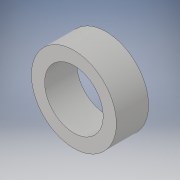
# Autodesk Inventor part: C-TFK10_c
Saved by Autodesk Inventor 2021 (Build 250183000, 183)
## iProperties
Created: 2023-03-01
Part Number: C-TFK10_c
Material: Generic
Catalog Web Link: www.cadenas.de
Description: C-TFK_c-Economy Support Units Fixed Side Round
Vendor: MISUMI
Document SubType Name: Modeling
Designer: psAdmin
Manufacturer: MISUMI
Mass: 0.476246 g
Surface Area: 5.9651 cm^2
Volume: 0.476246 cm^3
Density: 1 g/cm^3
Appearance: PSOLRGB-175-175-175
Category: PARTsolutions
Company: MISUMI
PSOL_IDENT_0: {$CADENAS_DATA/23d-libs/misumi/metric/09_ball_screws/c_tfk/c_tfk_collar.prj},161 {VTYP=3D},{NB=C-TFK
PSOL_IDENT_1: 10_c},{LINA=C-TFK10},{NN=C-TFK_c},{DATE=14.09.2022 01:48:01},{GEOMDATE=16.11.2021 00:24:26},{VERSION=
PSOL_IDENT_2: },{LINEID=100},{WBVAR=SET},{WBNUMERIC=}  {NB=C-TFK10_c},{LINA=C-TFK10},{KT=DUMMY},{PN=C-TFK10},{TYPE=
PSOL_IDENT_3: C-TFK},{NO=10},{SET=},{DD=10},{L=27},{H=10},{F=17},{E=29.5},{D=34},{A=52},{PCD=42},{B=42},{L1=7.5},{
PSOL_IDENT_4: T1=5.0},{DD1=4.5},{DD2=8.0},{LL=4.0},{M=M10x1.0},{T=16},{SID=14.0},{ACD=14.5},{ACV=10},{ACL=5.5}
NB: C-TFK10_c
NN: C-TFK_c
NT: Economy Support Units Fixed Side Round
NBSYN: $PN._c
LINA: C-TFK10
CATALOG: Misumi
PN: C-TFK10
NO: 10
SET: w/o SET
DD: 10
L: 27
H: 10
F: 17
E: 29.5
D: 34
A: 52
PCD: 42
B: 42
L1: 7.5
T1: 5
DD1: 4.5
DD2: 8
LL: 4
M: M10x1.0
T: 16
ACD: 14.5
ACV: 10
ACL: 5.5
SUPPLIER: MISUMI
ARTICLENO: C-TFK10_c
BOMINFO: C-TFK10
CREATOR: CADENAS GmbH
Title: C-TFK10
Author: Cadenas PARTsolutions
Comments: Economy Support Units Fixed Side Round
Autodesk Inventor part; units mm, degrees
sketch "Sketch_1" plane through (0, 0, 0) normal (0, 0, 1) x (1, 0, 0)
  circle A0 centre (0, 0) radius 7.25
  circle A1 centre (0, 0) radius 5
  constraints: 2 centre point
extrude "Extrusion1" add sketch "Sketch_1" along normal blind 5.5
ref_plane "to_base_XY" through (0, 0, 0) normal (0, 0, 1) x (1, 0, 0)
ref_plane "to_base_YZ" through (0, 0, 0) normal (1, 0, 0) x (0, 1, 0)
ref_plane "to_base_ZX" through (0, 0, 0) normal (0, 1, 0) x (0, 0, 1)
ref_plane "to_nut_XY" through (0, 0, 5.5) normal (0, 0, 1) x (1, 0, 0)
ref_plane "to_nut_YZ" through (0, 0, 5.5) normal (1, 0, 0) x (0, 1, 0)
ref_plane "to_nut_ZX" through (0, 0, 5.5) normal (0, 1, 0) x (0, 0, 1)
body "Solid1"
